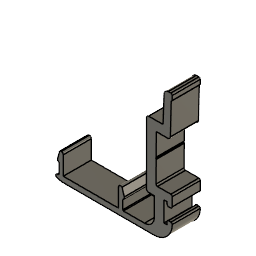
Traslape (Autodesk Fusion 360 design; units mm, degrees)
part number: 2025-12-28-14-21-04-778
Autodesk Fusion 360 part; units mm, degrees
sketch "Boceto1" plane through (0, 0, 0) normal (0, 1, 0) x (1, 0, 0)
  line L0 (2.6809, 0) -> (34.86, 0)
  arc A0 (41.36, -6.5) -> (34.86, 0) centre (34.86, -6.5) ccw
  line L1 (40.86, -46.76) -> (39.9461, -46.7599)
  line L2 (38.4472, -45.3141) -> (38.1117, -36.0373)
  line L3 (37.7619, -35.7) -> (32.95, -35.7)
  line L4 (32.2, -34.95) -> (32.2, -12.95)
  line L5 (32.95, -12.2) -> (35, -12.2)
  line L6 (35, -12.2) -> (35, -5.5)
  arc A1 (35, -5.5) -> (31.5, -2) centre (31.5, -5.5) ccw
  arc A2 (32.95, -12.2) -> (32.2, -12.95) centre (32.95, -12.95) ccw
  arc A3 (32.2, -34.95) -> (32.95, -35.7) centre (32.95, -34.95) ccw
  arc A4 (38.4472, -45.3141) -> (39.9461, -46.7599) centre (39.9462, -45.2599) ccw
  arc A5 (40.86, -46.76) -> (41.36, -46.26) centre (40.86, -46.26) ccw
  arc A6 (38.1117, -36.0373) -> (37.7619, -35.7) centre (37.7619, -36.05) ccw
  line L7 (40.86, -7) -> (40, -7)
  line L8 (39.5, -6.5) -> (39.5, -5.5)
  line L9 (39.5, -5.5) -> (38.4, -5.5)
  line L10 (38.4, -5.5) -> (38.4, -12.6)
  line L11 (38.4, -12.6) -> (39.5, -12.6)
  line L12 (39.5, -12.6) -> (39.5, -11.95)
  line L13 (40.15, -11.3) -> (40.71, -11.3)
  arc A7 (40.15, -11.3) -> (39.5, -11.95) centre (40.15, -11.95) ccw
  arc A8 (41.36, -11.95) -> (40.71, -11.3) centre (40.71, -11.95) ccw
  arc A9 (39.5, -6.5) -> (40, -7) centre (40, -6.5) ccw
  arc A10 (40.86, -7) -> (41.36, -6.5) centre (40.86, -6.5) ccw
  line L14 (40.86, -15.6) -> (36.103, -15.6)
  line L15 (35.7, -32.3) -> (39.7578, -32.2757)
  line L16 (40.7132, -33.2016) -> (40.9951, -44.3051)
  line L17 (41.195, -44.5) -> (41.16, -44.5)
  line L18 (41.36, -11.95) -> (41.36, -15.1)
  line L19 (41.36, -44.7) -> (41.36, -46.26)
  arc A11 (41.36, -44.7) -> (41.16, -44.5) centre (41.16, -44.7) ccw
  arc A12 (40.9951, -44.3051) -> (41.195, -44.5) centre (41.195, -44.3) ccw
  arc A13 (40.7132, -33.2016) -> (39.7578, -32.2757) centre (39.7635, -33.2257) ccw
  line L20 (35.45, -24.05) -> (35.5469, -23.9524)
  line L21 (35.45, -24.05) -> (35.5481, -24.1464)
  line L22 (35.603, -16.103) -> (35.6485, -23.7037)
  line L23 (35.6527, -24.3939) -> (35.7, -32.3)
  arc A14 (35.6527, -24.3939) -> (35.5481, -24.1464) centre (35.3027, -24.396) ccw
  arc A15 (35.5469, -23.9524) -> (35.6485, -23.7037) centre (35.2985, -23.7058) ccw
  arc A16 (40.86, -15.6) -> (41.36, -15.1) centre (40.86, -15.1) ccw
  arc A17 (36.103, -15.6) -> (35.603, -16.103) centre (36.103, -16.1) ccw
  line L24 (22.25, -2.25) -> (22.25, -8.55)
  line L25 (23.75, -2.25) -> (23.75, -5.4262)
  arc A18 (22.25, -8.55) -> (23, -9.3) centre (23, -8.55) ccw
  arc A19 (23, -9.3) -> (23.5303, -9.0803) centre (23, -8.55) ccw
  line L26 (23.5303, -9.0803) -> (24.2979, -6.4837)
  line L27 (23.8619, -5.482) -> (23.75, -5.4262)
  arc A20 (24.2979, -6.4837) -> (23.8619, -5.482) centre (23.4828, -6.2427) ccw
  line L28 (31.5, -2) -> (24, -2)
  arc A21 (22.25, -2.25) -> (22, -2) centre (22, -2.25) ccw
  arc A22 (24, -2) -> (23.75, -2.25) centre (24, -2.25) ccw
  line L29 (1.1, -2) -> (1.1, -5.4752)
  line L30 (1.8, -9.3) -> (1.9, -9.3)
  line L31 (2.6, -8.6) -> (2.6, -2)
  arc A23 (1.9, -9.3) -> (2.6, -8.6) centre (1.9, -8.6) ccw
  arc A24 (1.2908, -9.0803) -> (1.8, -9.3) centre (1.8, -8.6) ccw
  line L32 (2.6807, -9.0803) -> (0.7719, -9.0803) construction
  line L33 (2.395, -9.095) -> (24.5, -5.8) construction
  line L34 (24.5, -5.8) -> (0, -5.8) construction
  line L35 (1.305, -9.095) -> (0.5905, -6.4934)
  line L36 (23.75, -5.4262) -> (-2.0557, -5.482) construction
  line L37 (1.0523, -5.4973) -> (1.1, -5.4752)
  arc A25 (1.0523, -5.4973) -> (0.5905, -6.4934) centre (1.4101, -6.2683) ccw
  line L38 (22, -2) -> (2.6, -2)
  line L39 (1.1, -2) -> (1.1001, -1.9004)
  line L40 (0.5009, -1.65) -> (0.8503, -1.6502)
  arc A26 (1.1001, -1.9004) -> (0.8503, -1.6502) centre (0.8501, -1.9002) ccw
  line L41 (0.3324, -0.4739) -> (0.4057, -0.4441)
  arc A27 (2.6809, 0) -> (0.4057, -0.4441) centre (2.6809, -6.05) ccw
  arc A28 (0.3324, -0.4739) -> (0.5009, -1.65) centre (0.5014, -1.0498) ccw
  point P0 (41.36, 0)
  point P1 (41.36, -46.76)
  point P2 (2.6, -9.3)
  dimension "d1" = 41.36
  dimension "d2" = 46.76
  dimension "d3" = 6.5
  dimension "d4" = 3.5
  dimension "d5" = 0.75
  dimension "d6" = 0.75
  dimension "d7" = 1.5
  dimension "d8" = 0.5
  dimension "d9" = 0.35
  dimension "d10" = 0.65
  dimension "d11" = 0.5
  dimension "d12" = 0.2
  dimension "d13" = 0.95
  dimension "d16" = 0.35
  dimension "d17" = 0.5
  dimension "d18" = 0.75
  dimension "d19" = 0.85
  dimension "d20" = 0.25
  dimension "d24" = 7.3
  dimension "d25" = 1.5
  dimension "d26" = 0.7
  dimension "d27" = 0.85
  dimension "d28" = 0.25
  dimension "d29" = 6.05
  constraint horizontal L0
  constraint coincident P0 L0
  constraint tangent L0 A0
  constraint perpendicular L3 L4
  constraint perpendicular L4 L5
  constraint perpendicular L5 L6
  constraint perpendicular L6 L28
  constraint tangent L6 A1
  constraint tangent A1 L28
  constraint tangent L4 A2
  constraint tangent L5 A2
  constraint tangent L3 A3
  constraint tangent L4 A3
  constraint tangent L1 A4
  constraint tangent L2 A4
  constraint coincident P1 L1
  constraint tangent L1 A5
  constraint tangent L2 A6
  constraint tangent L3 A6
  constraint perpendicular L7 L8
  constraint perpendicular L8 L9
  constraint perpendicular L9 L10
  constraint perpendicular L10 L11
  constraint perpendicular L11 L12
  constraint tangent L12 A7
  constraint tangent L13 A7
  constraint tangent L13 A8
  constraint tangent A8 L18
  constraint equal A7 A8
  constraint tangent L7 A9
  constraint tangent L8 A9
  constraint tangent L7 A10
  constraint equal A9 A10
  constraint coincident A0.start A10.end
  constraint perpendicular L14 L18
  constraint perpendicular L15 L22
  constraint perpendicular L17 L18
  constraint collinear L18 L19
  constraint tangent L17 A11
  constraint tangent L19 A11
  constraint tangent L16 A12
  constraint tangent L17 A12
  constraint equal A11 A12
  constraint tangent L15 A13
  constraint tangent L16 A13
  constraint collinear L22 L23
  constraint tangent L21 A14
  constraint tangent L23 A14
  constraint tangent L20 A15
  constraint tangent L22 A15
  constraint equal A14 A15
  constraint tangent L14 A16
  constraint tangent L18 A16
  constraint tangent L14 A17
  constraint tangent L22 A17
  constraint equal A16 A17
  constraint perpendicular L24 L28
  constraint perpendicular L25 L28
  constraint tangent L24 A18
  constraint tangent L25 A19
  constraint equal A18 A19
  constraint coincident A18.end A19.start
  constraint tangent L26 A20
  constraint tangent L27 A20
  constraint collinear L28 L38
  constraint tangent L24 A21
  constraint tangent A21 L38
  constraint tangent L25 A22
  constraint tangent L28 A22
  constraint equal A21 A22
  constraint vertical L29
  constraint horizontal L30
  constraint vertical L31
  constraint coincident P2 L30
  constraint coincident P2 L31
  constraint tangent L30 A23
  constraint tangent L31 A23
  constraint tangent L29 A24
  constraint tangent L30 A24
  constraint equal A23 A24
  constraint perpendicular L25 L32
  constraint midpoint A23 L33.start
  constraint perpendicular L29 L34
  constraint coincident L32 A24.start
  constraint coincident A24 L35.start
  constraint coincident L36 L29.end
  constraint tangent L35 A25
  constraint tangent L37 A25
  constraint tangent L40 A28
  constraint perpendicular L39 L40
  constraint tangent L40 A26
  constraint tangent L39 A26
  constraint tangent L41 A27
  constraint tangent L0 A27
  measures "d1" distance of origin P0
  measures "d2" distance of P0 P1
  measures "d3" radius of A0
  measures "d4" radius of A1
  measures "d5" radius of A2
  measures "d6" radius of A3
  measures "d7" radius of A4
  measures "d8" radius of A5
  measures "d9" radius of A6
  measures "d10" radius of A7
  measures "d11" radius of A9
  measures "d12" radius of A11
  measures "d13" radius of A13
  measures "d16" radius of A14
  measures "d17" radius of A16
  measures "d18" radius of A18
  measures "d19" radius of A20
  measures "d20" radius of A21
  measures "d24" distance of L31.end P2
  measures "d25" distance of L29 L31
  measures "d26" radius of A23
  measures "d27" radius of A25
  measures "d28" radius of A26
  measures "d29" radius of A27
extrude "Extruir1" add sketch "Boceto1" along normal blind 10
equation "L = 10 mm"
equation "d31 = L"
